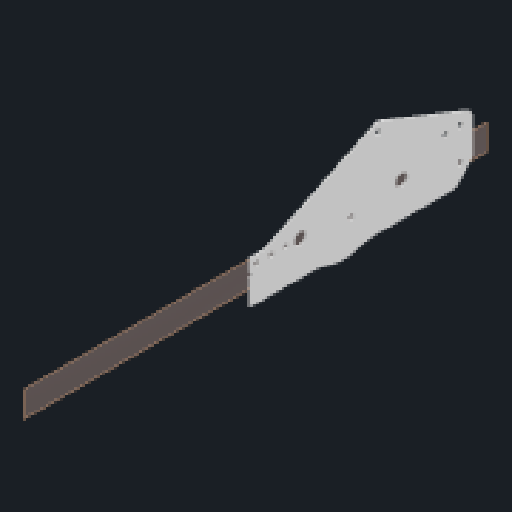
# Autodesk Inventor part: Part161
Saved by Autodesk Inventor 2025 (Build 290162010, 162A)
## iProperties
Created: 2025-10-28
Part Number: Part161
Material: Generic
Document SubType Name: Modeling
Designer: jasper
Density: 1 g/cm^3
Appearance: Default
Author: jasper
Autodesk Inventor part; units mm, degrees
ref_plane "YZ Plane" through (0, 0, 0) normal (1, 0, 0) x (0, 1, 0)
ref_plane "XZ Plane" through (0, 0, 0) normal (0, 1, 0) x (-1, 0, 0)
ref_plane "XY Plane" through (0, 0, 0) normal (0, 0, 1) x (1, 0, 0)
ref_plane "Work Plane1" through (-72.8386, -105.7169, -152.268) normal (1, 0, 0) x (0, 1, 0)
sketch "Sketch1" plane through (-72.8386, -105.7169, -152.268) normal (1, 0, 0) x (0, 1, 0)
  line L0 (-41.2196, 6.35) -> (64.7019, 6.35)
  circle A0 centre (0, 6.35) radius 2.1844
  line L1 (-12.7, -5.2578) -> (-12.7, 56.2102) projected
  line L2 (-24.13, 6.35) -> (-24.13, -171.3455)
  line L3 (-22.1107, -175.9896) -> (-9.7415, -187.5241)
  line L4 (-5.4108, -189.23) -> (23.8328, -189.23)
  circle A1 centre (52.4757, -106.725) radius 2.1844 projected
  line L5 (12.7, 56.2102) -> (12.7, -5.2578) projected
  circle A2 centre (52.4757, -106.725) radius 7.62
  line L6 (2.3114, -184.15) -> (10.3188, -184.15) projected
  line L7 (-12.7, -184.15) -> (-12.7, -134.2898) projected
  line L8 (59.5652, -109.5185) -> (29.7407, -185.2079)
  line L9 (-24.13, 5.842) -> (67.0388, 5.842)
  line L10 (59.3372, -103.4107) -> (15.2284, -12.0924)
  line L11 (12.7, -1.0449) -> (12.7, 5.842)
  circle A3 centre (21.8059, -177.8) radius 2.1844 projected
  circle A4 centre (21.8059, -165.1) radius 2.1844 projected
  circle A5 centre (-6.35, -76.2) radius 2.1844 projected
  circle A6 centre (-6.35, -76.2) radius 20.32
  line L12 (-24.13, -50.8) -> (-24.13, -63.5) construction
  line L13 (-24.13, -63.5) -> (-36.83, -76.2) construction
  line L14 (-36.83, -76.2) -> (-24.13, -88.9) construction
  line L15 (-24.13, -88.9) -> (-24.13, -101.6) construction
  spline S0 degree 4 poles (-24.13, -50.8) (-24.13, -63.5) (-36.83, -76.2) (-24.13, -88.9) (-24.13, -101.6) knots 1 1 1 1 1 2 2 2 2 2
  arc A7 (12.7, -1.0449) -> (15.2284, -12.0924) centre (38.1, -1.0449) ccw
  arc A8 (23.8328, -189.23) -> (29.7407, -185.2079) centre (23.8328, -182.88) ccw
  arc A9 (-9.7415, -187.5241) -> (-5.4108, -189.23) centre (-5.4108, -182.88) ccw
  arc A10 (-24.13, -171.3455) -> (-22.1107, -175.9896) centre (-17.78, -171.3455) ccw
  circle A11 centre (6.35, -38.1) radius 2.1844
  circle A12 centre (6.35, -38.1) radius 5.08
  circle A13 centre (6.35, -127) radius 2.1844
  circle A14 centre (6.35, -127) radius 5.08
  circle A15 centre (0, -82.55) radius 2.1844
  line L16 (10.3187, 184.15) -> (-10.3187, 184.15) projected
  circle A16 centre (6.35, -25.4) radius 2.1844 projected
  circle A17 centre (6.35, -12.7) radius 2.1844 projected
  circle A18 centre (6.35, 0) radius 2.1844 projected
  circle A19 centre (-6.35, -177.8) radius 2.1844 projected
  circle A20 centre (0, -6.35) radius 2.1844
  circle A21 centre (0, -19.05) radius 2.1844
  point P0 (105.7169, 152.268)
  point P1 (-7.9121, -189.23)
  point P2 (28.1559, -189.23)
  point P3 (12.7, -6.858)
  point P4 (12.7, -1.0449)
  point P5 (12.7, 5.842)
  point P6 (2.1245, 5.842)
  point P7 (-2.1245, 5.842)
  point P8 (-24.13, -66.3626)
  point P9 (-24.13, -86.0374)
  dimension "d0" = 15.24
  dimension "d1" = 5.08
  dimension "d3" = 11.43
  dimension "d4" = 133
  dimension "d5" = 40.64
  dimension "d6" = 6.35
  dimension "d7" = 36.068
  dimension "d8" = 0.508
  dimension "d9" = 12.7
  dimension "d10" = 12.7
  dimension "d11" = 12.7
  dimension "d12" = 12.7
  dimension "d13" = 12.7
  dimension "d14" = 12.7
  dimension "d15" = 25.4
  dimension "d16" = 6.35
  dimension "d17" = 10.16
  dimension "d18" = 10.16
  dimension "d21" = 12.7
  dimension "d22" = 12.7
  dimension "d23" = 4.3688
  dimension "d24" = 4.3688
  constraints: 16 end point, 14 centre point, 13 point on line, 10 point on circle, 10 tangent, 4 coincident, 3 perpendicular, 2 equal radius, 2 vertical, 2 vertical alignment, 1 horizontal, 1 horizontal alignment, 1 parallel, 11 other
  measures "d0" diameter of A2
  measures "d1" distance between parallel lines of L6 L4
  measures "d3" distance between parallel lines of L7 L2
  measures "d4" angle of L2 L3
  measures "d5" diameter of A6
  measures "d6" horizontal distance of A3.centre point (28.156, -189.23)
  measures "d7" distance of point (-7.912, -189.23) point (28.156, -189.23)
  measures "d8" distance between parallel lines of L0 L9
  measures "d9" distance of point (12.7, -6.858) L11.end
  measures "d10" horizontal distance of L12.end L13.end
  measures "d11" horizontal distance of L13.end L14.end
  measures "d12" distance from line of L2 L13.end
  measures "d13" distance of L15.end L14.end
  measures "d14" distance of L12.start L12.end
  measures "d15" radius of A7
  measures "d16" radius of A8
  measures "d17" diameter of A12
  measures "d18" diameter of A14
  measures "d21" distance of A0.centre A20.centre
  measures "d22" distance of A20.centre A21.centre
  measures "d23" diameter of A21
  measures "d24" diameter of A20
extrude "Extrusion1" add sketch "Sketch1" along normal blind 1.5875 contours L9 A0 L5 A7 L10 A2 L8 A8 L4 A9 L3 A10 L2 A6 | L2 A6 S0 | A6 L2 | L2 A6 | A2 | A15 | A16 | A17 | A18
body "Solid1"
